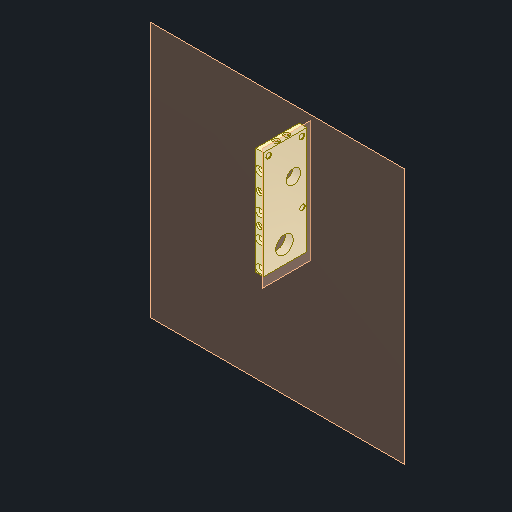
# Autodesk Inventor part: left_gear_holder
Saved by Autodesk Inventor 2023 (Build 270158000, 158)
## iProperties
Created: 2024-04-23
Part Number: left_gear_holder
Material: Nylon 6/6
Document SubType Name: Modeling
Designer: szymo
Density: 1.13 g/cm^3
Appearance: Nylon 6
Mass: 14.9327 g
Surface Area: 88.4291 cm^2
Volume: 13.2148 cm^3
Author: szymo
Autodesk Inventor part; units mm, degrees
ref_plane "YZ Plane" through (0, 0, 0) normal (1, 0, 0) x (0, 1, 0)
ref_plane "XZ Plane" through (0, 0, 0) normal (0, 1, 0) x (-1, 0, 0)
ref_plane "XY Plane" through (0, 0, 0) normal (0, 0, 1) x (1, 0, 0)
ref_plane "Work Plane1" through (0, 0, 0) normal (0, 0, 1) x (1, 0, 0)
sketch "Sketch1" plane through (0, 0, 0) normal (0, 0, 1) x (1, 0, 0)
  line L0 (23.5, 88.5) -> (-23.5, 88.5) projected
  line L1 (-23.5, 88.5) -> (-23.5, 36.5) projected
  line L2 (-26.5, 33.5) -> (-89, 33.5) projected
  line L3 (-89, 33.5) -> (-89, -72.5) projected
  line L4 (-89, -72.5) -> (-77, -72.5) projected
  line L5 (-74, -75.5) -> (-74, -93.5) projected
  line L6 (-74, -93.5) -> (74, -93.5) projected
  line L7 (74, -93.5) -> (74, -75.5) projected
  line L8 (77, -72.5) -> (89, -72.5) projected
  line L9 (89, -72.5) -> (89, 33.5) projected
  line L10 (89, 33.5) -> (26.5, 33.5) projected
  line L11 (23.5, 36.5) -> (23.5, 88.5) projected
  line L12 (-4.5, 81.5) -> (-4.5, 36.5) projected
  line L13 (-7.5, 33.5) -> (-13.5, 33.5) projected
  line L14 (-16.5, 36.5) -> (-16.5, 81.5) projected
  line L15 (-13.5, 84.5) -> (-7.5, 84.5) projected
  line L16 (16.5, 81.5) -> (16.5, 36.5) projected
  line L17 (13.5, 33.5) -> (7.5, 33.5) projected
  line L18 (4.5, 36.5) -> (4.5, 81.5) projected
  line L19 (7.5, 84.5) -> (13.5, 84.5) projected
  line L20 (16.5, 88.5) -> (22.5, 88.5)
  line L21 (22.5, 88.5) -> (22.5, 3.75)
  line L22 (22.5, 3.75) -> (16.5, 3.75)
  line L23 (16.5, 3.75) -> (16.5, 88.5)
  line L24 (59.9, 4.75) -> (32.2, 4.75)
  arc A0 (13.5, 33.5) -> (16.5, 36.5) centre (13.5, 36.5) ccw projected
  arc A1 (4.5, 36.5) -> (7.5, 33.5) centre (7.5, 36.5) ccw projected
  arc A2 (7.5, 84.5) -> (4.5, 81.5) centre (7.5, 81.5) ccw projected
  arc A3 (16.5, 81.5) -> (13.5, 84.5) centre (13.5, 81.5) ccw projected
  arc A4 (-4.5, 81.5) -> (-7.5, 84.5) centre (-7.5, 81.5) ccw projected
  arc A5 (-7.5, 33.5) -> (-4.5, 36.5) centre (-7.5, 36.5) ccw projected
  arc A6 (-16.5, 36.5) -> (-13.5, 33.5) centre (-13.5, 36.5) ccw projected
  arc A7 (-13.5, 84.5) -> (-16.5, 81.5) centre (-13.5, 81.5) ccw projected
  arc A8 (-26.5, 33.5) -> (-23.5, 36.5) centre (-26.5, 36.5) ccw projected
  arc A9 (-74, -75.5) -> (-77, -72.5) centre (-77, -75.5) ccw projected
  arc A10 (77, -72.5) -> (74, -75.5) centre (77, -75.5) ccw projected
  arc A11 (23.5, 36.5) -> (26.5, 33.5) centre (26.5, 36.5) ccw projected
  circle A12 centre (39.125, 25.9125) radius 1.0065 projected
  circle A13 centre (72.95, 12.275) radius 1.0065 projected
  circle A14 centre (-39.125, 12.3375) radius 1.0065 projected
  circle A15 centre (-72.95, 25.975) radius 1.0065 projected
  circle A16 centre (-72.95, 12.275) radius 1.0065 projected
  circle A17 centre (-39.125, 25.9125) radius 1.0065 projected
  circle A18 centre (72.95, 25.975) radius 1.0065 projected
  circle A19 centre (39.125, 12.3375) radius 1.0065 projected
  circle A20 centre (-42.4984, -44.6666) radius 1.2295 projected
  circle A21 centre (-79, -42.3889) radius 1.2295 projected
  circle A22 centre (-19.5, 28.875) radius 1.2295 projected
  circle A23 centre (19.5, 9.55) radius 1.2295 projected
  circle A24 centre (19.5, 47.3) radius 1.2295 projected
  circle A25 centre (-19.5, 47.3) radius 1.2295 projected
  circle A26 centre (0, 74.7) radius 1.2295 projected
  circle A27 centre (-19.4231, 74.8077) radius 1.2295 projected
  circle A28 centre (19.5, 74.7) radius 1.2295 projected
  circle A29 centre (0, 49.05) radius 1.2295 projected
  circle A30 centre (19.5, 28.875) radius 1.2295 projected
  circle A31 centre (0, 19.125) radius 1.2295 projected
  circle A32 centre (-19.5, 9.55) radius 1.2295 projected
  circle A33 centre (42.5, -44.6649) radius 1.2295 projected
  circle A34 centre (79, -42.3889) radius 1.2295 projected
  circle A35 centre (21.5, -85.5) radius 1.8 projected
  circle A36 centre (-64.5, -85.5) radius 1.8 projected
  circle A37 centre (-21.5, -85.5) radius 1.8 projected
  circle A38 centre (64.5, -85.5) radius 1.8 projected
  line L25 (-58.2315, -77.6013) -> (-80.7685, -61.1541) projected
  line L26 (-82, -58.7308) -> (-82, -48.3889) projected
  line L27 (-75.8885, -45.3972) -> (-47.1423, -47.5438) projected
  line L28 (-21.1, -26.5751) -> (-21.1, -22.0813) projected
  line L29 (-46.9357, -41.5592) -> (-76, -39.3889) projected
  line L30 (-82, -36.3889) -> (-82, 1.75) projected
  line L31 (32.9914, 4.75) -> (79, 4.75) projected
  line L32 (82, -48.3889) -> (82, -58.7308) projected
  line L33 (76, -39.3889) -> (46.9371, -41.5577) projected
  line L34 (21.1, -22.0813) -> (21.1, -26.5749) projected
  line L35 (47.144, -47.5423) -> (76, -45.3889) projected
  line L36 (82, 1.75) -> (82, -36.3889) projected
  line L37 (80.7685, -61.1541) -> (58.2315, -77.6013) projected
  line L38 (57, -80.0246) -> (57, -87.5) projected
  arc A39 (55, -89.5) -> (57, -87.5) centre (55, -87.5) ccw projected
  line L39 (55, -89.5) -> (31, -89.5) projected
  arc A40 (29, -87.5) -> (31, -89.5) centre (31, -87.5) ccw projected
  line L40 (29, -87.5) -> (29, -79.2522) projected
  line L41 (14, -79.5039) -> (14, -87.5) projected
  arc A41 (12, -89.5) -> (14, -87.5) centre (12, -87.5) ccw projected
  line L42 (12, -89.5) -> (-12, -89.5) projected
  arc A42 (-14, -87.5) -> (-12, -89.5) centre (-12, -87.5) ccw projected
  line L43 (-14, -87.5) -> (-14, -79.5039) projected
  line L44 (-29, -79.2522) -> (-29, -87.5) projected
  arc A43 (-31, -89.5) -> (-29, -87.5) centre (-31, -87.5) ccw projected
  line L45 (-31, -89.5) -> (-55, -89.5) projected
  arc A44 (-57, -87.5) -> (-55, -89.5) centre (-55, -87.5) ccw projected
  line L46 (-57, -87.5) -> (-57, -80.0246) projected
  line L47 (-66.95, 28.9125) -> (-45.125, 28.9125) projected
  line L48 (-42.125, 25.9125) -> (-42.125, 12.275) projected
  line L49 (-45.125, 9.275) -> (-66.95, 9.275) projected
  line L50 (-69.95, 12.275) -> (-69.95, 25.9125) projected
  line L51 (-16.5, 12.75) -> (-16.5, 25.5) projected
  line L52 (-13.5, 28.5) -> (-7.5, 28.5) projected
  line L53 (-4.5, 25.5) -> (-4.5, 12.75) projected
  line L54 (-7.5, 9.75) -> (-13.5, 9.75) projected
  line L55 (66.95, 9.3375) -> (45.125, 9.3375) projected
  line L56 (42.125, 12.3375) -> (42.125, 25.975) projected
  line L57 (45.125, 28.975) -> (66.95, 28.975) projected
  line L58 (69.95, 25.975) -> (69.95, 12.3375) projected
  line L59 (4.5, 12.75) -> (4.5, 25.5) projected
  line L60 (7.5, 28.5) -> (13.5, 28.5) projected
  line L61 (16.5, 25.5) -> (16.5, 12.75) projected
  line L62 (13.5, 9.75) -> (7.5, 9.75) projected
  line L63 (44.5181, -40.6102) -> (28.0504, -22.9209) projected
  line L64 (27.268, -20.5154) -> (30.0132, 2.1113) projected
  line L65 (-44.7206, -49.1201) -> (-29.3549, -77.8368) projected
  line L66 (-79, 4.75) -> (-32.9914, 4.75) projected
  line L67 (-30.0132, 2.1113) -> (-27.268, -20.5155) projected
  line L68 (-28.0502, -22.9208) -> (-44.5164, -40.6115) projected
  line L69 (29.3549, -77.8368) -> (44.7222, -49.1185) projected
  line L70 (-14.6042, -77.6983) -> (-37.8537, -46.8489) projected
  line L71 (-37.4786, -42.8259) -> (-22.0793, -28.7924) projected
  line L72 (-21.1218, -21.72) -> (-23.9255, 1.3887) projected
  line L73 (-20.9474, 4.75) -> (20.9474, 4.75) projected
  line L74 (23.9255, 1.3887) -> (21.1218, -21.72) projected
  line L75 (22.0795, -28.7925) -> (37.4798, -42.8243) projected
  line L76 (37.8551, -46.8475) -> (14.6042, -77.6983) projected
  circle A45 centre (-78, -67.1725) radius 1.2295 projected
  arc A46 (79, -39.3889) -> (82, -36.3889) centre (79, -36.3889) ccw projected
  arc A47 (44.5181, -40.6102) -> (46.9371, -41.5577) centre (46.7138, -38.566) ccw projected
  arc A48 (27.268, -20.5154) -> (28.0504, -22.9209) centre (30.2461, -20.8767) ccw projected
  arc A49 (32.9914, 4.75) -> (30.0132, 2.1113) centre (32.9914, 1.75) ccw projected
  arc A50 (82, 1.75) -> (79, 4.75) centre (79, 1.75) ccw projected
  arc A51 (-42.125, 25.9125) -> (-45.125, 28.9125) centre (-45.125, 25.9125) ccw projected
  arc A52 (-45.125, 9.275) -> (-42.125, 12.275) centre (-45.125, 12.275) ccw projected
  arc A53 (-69.95, 12.275) -> (-66.95, 9.275) centre (-66.95, 12.275) ccw projected
  arc A54 (-66.95, 28.9125) -> (-69.95, 25.9125) centre (-66.95, 25.9125) ccw projected
  arc A55 (-13.5, 28.5) -> (-16.5, 25.5) centre (-13.5, 25.5) ccw projected
  arc A56 (-4.5, 25.5) -> (-7.5, 28.5) centre (-7.5, 25.5) ccw projected
  arc A57 (-7.5, 9.75) -> (-4.5, 12.75) centre (-7.5, 12.75) ccw projected
  arc A58 (-16.5, 12.75) -> (-13.5, 9.75) centre (-13.5, 12.75) ccw projected
  arc A59 (58.2315, -77.6013) -> (57, -80.0246) centre (60, -80.0246) ccw projected
  arc A60 (29.3549, -77.8368) -> (29, -79.2522) centre (32, -79.2522) ccw projected
  arc A61 (47.144, -47.5423) -> (44.7222, -49.1185) centre (47.3673, -50.5339) ccw projected
  arc A62 (82, -48.3889) -> (79, -45.3889) centre (79, -48.3889) ccw projected
  arc A63 (80.7685, -61.1541) -> (82, -58.7308) centre (79, -58.7308) ccw projected
  arc A64 (-21.1, -22.0813) -> (-21.1218, -21.72) centre (-24.1, -22.0813) ccw projected
  arc A65 (-20.9474, 4.75) -> (-23.9255, 1.3887) centre (-20.9474, 1.75) ccw projected
  arc A66 (23.9255, 1.3887) -> (20.9474, 4.75) centre (20.9474, 1.75) ccw projected
  arc A67 (21.1218, -21.72) -> (21.1, -22.0813) centre (24.1, -22.0813) ccw projected
  arc A68 (21.1, -26.5749) -> (22.0795, -28.7925) centre (24.1, -26.5749) ccw projected
  arc A69 (37.8551, -46.8475) -> (37.4798, -42.8243) centre (35.4593, -45.0419) ccw projected
  arc A70 (14.6042, -77.6983) -> (14, -79.5039) centre (17, -79.5039) ccw projected
  arc A71 (-14, -79.5039) -> (-14.6042, -77.6983) centre (-17, -79.5039) ccw projected
  arc A72 (-37.4786, -42.8259) -> (-37.8537, -46.8489) centre (-35.4579, -45.0433) ccw projected
  arc A73 (-22.0793, -28.7924) -> (-21.1, -26.5751) centre (-24.1, -26.5751) ccw projected
  arc A74 (-82, -36.3889) -> (-79, -39.3889) centre (-79, -36.3889) ccw projected
  arc A75 (-79, 4.75) -> (-82, 1.75) centre (-79, 1.75) ccw projected
  arc A76 (-30.0132, 2.1113) -> (-32.9914, 4.75) centre (-32.9914, 1.75) ccw projected
  arc A77 (-28.0502, -22.9208) -> (-27.268, -20.5155) centre (-30.2461, -20.8769) ccw projected
  arc A78 (-46.9357, -41.5592) -> (-44.5164, -40.6115) centre (-46.7123, -38.5676) ccw projected
  arc A79 (7.5, 28.5) -> (4.5, 25.5) centre (7.5, 25.5) ccw projected
  arc A80 (16.5, 25.5) -> (13.5, 28.5) centre (13.5, 25.5) ccw projected
  arc A81 (13.5, 9.75) -> (16.5, 12.75) centre (13.5, 12.75) ccw projected
  arc A82 (4.5, 12.75) -> (7.5, 9.75) centre (7.5, 12.75) ccw projected
  arc A83 (-57, -80.0246) -> (-58.2315, -77.6013) centre (-60, -80.0246) ccw projected
  arc A84 (-82, -58.7308) -> (-80.7685, -61.1541) centre (-79, -58.7308) ccw projected
  arc A85 (-75.8885, -45.3972) -> (-76.1119, -45.3889) centre (-76.1119, -48.3889) ccw projected
  arc A86 (-44.7206, -49.1201) -> (-47.1423, -47.5438) centre (-47.3657, -50.5355) ccw projected
  arc A87 (-29, -79.2522) -> (-29.3549, -77.8368) centre (-32, -79.2522) ccw projected
  arc A88 (42.125, 12.3375) -> (45.125, 9.3375) centre (45.125, 12.3375) ccw projected
  arc A89 (45.125, 28.975) -> (42.125, 25.975) centre (45.125, 25.975) ccw projected
  arc A90 (69.95, 25.975) -> (66.95, 28.975) centre (66.95, 25.975) ccw projected
  arc A91 (66.95, 9.3375) -> (69.95, 12.3375) centre (66.95, 12.3375) ccw projected
  circle A92 centre (78, -67.1725) radius 1.2295 projected
  line L77 (-22.5, 25.9125) -> (-22.5, 12.55) projected
  arc A93 (-25.5, 9.55) -> (-22.5, 12.55) centre (-25.5, 12.55) ccw projected
  line L78 (-25.5, 9.55) -> (-33.125, 9.55) projected
  arc A94 (-36.125, 12.55) -> (-33.125, 9.55) centre (-33.125, 12.55) ccw projected
  line L79 (-36.125, 12.55) -> (-36.125, 25.9125) projected
  arc A95 (-33.125, 28.9125) -> (-36.125, 25.9125) centre (-33.125, 25.9125) ccw projected
  line L80 (-33.125, 28.9125) -> (-25.5, 28.9125) projected
  arc A96 (-22.5, 25.9125) -> (-25.5, 28.9125) centre (-25.5, 25.9125) ccw projected
  line L81 (76, -45.3889) -> (79, -45.3889) projected
  line L82 (79, -39.3889) -> (76, -39.3889) projected
  line L83 (33.125, 9.275) -> (25.5, 9.275) projected
  arc A97 (22.5, 12.275) -> (25.5, 9.275) centre (25.5, 12.275) ccw projected
  line L84 (22.5, 12.275) -> (22.5, 25.9125) projected
  arc A98 (25.5, 28.9125) -> (22.5, 25.9125) centre (25.5, 25.9125) ccw projected
  line L85 (25.5, 28.9125) -> (33.125, 28.9125) projected
  arc A99 (36.125, 25.9125) -> (33.125, 28.9125) centre (33.125, 25.9125) ccw projected
  line L86 (36.125, 25.9125) -> (36.125, 12.275) projected
  arc A100 (33.125, 9.275) -> (36.125, 12.275) centre (33.125, 12.275) ccw projected
  line L87 (-83, 28.975) -> (-78.95, 28.975) projected
  arc A101 (-75.95, 25.975) -> (-78.95, 28.975) centre (-78.95, 25.975) ccw projected
  line L88 (-75.95, 25.975) -> (-75.95, 12.275) projected
  arc A102 (-78.95, 9.275) -> (-75.95, 12.275) centre (-78.95, 12.275) ccw projected
  line L89 (-78.95, 9.275) -> (-83, 9.275) projected
  arc A103 (-86, 12.275) -> (-83, 9.275) centre (-83, 12.275) ccw projected
  line L90 (-86, 12.275) -> (-86, 25.975) projected
  arc A104 (-83, 28.975) -> (-86, 25.975) centre (-83, 25.975) ccw projected
  arc A105 (-79, -45.3889) -> (-82, -48.3889) centre (-79, -48.3889) ccw projected
  line L91 (-79, -45.3889) -> (-76.1119, -45.3889) projected
  line L92 (-76, -39.3889) -> (-79, -39.3889) projected
  line L93 (78.95, 28.975) -> (83, 28.975) projected
  arc A106 (86, 25.975) -> (83, 28.975) centre (83, 25.975) ccw projected
  line L94 (86, 25.975) -> (86, 12.275) projected
  arc A107 (83, 9.275) -> (86, 12.275) centre (83, 12.275) ccw projected
  line L95 (83, 9.275) -> (78.95, 9.275) projected
  arc A108 (75.95, 12.275) -> (78.95, 9.275) centre (78.95, 12.275) ccw projected
  line L96 (75.95, 12.275) -> (75.95, 25.975) projected
  arc A109 (78.95, 28.975) -> (75.95, 25.975) centre (78.95, 25.975) ccw projected
  circle A110 centre (-24.1, -73.1) radius 1.2295 projected
  circle A111 centre (24.1, -24.9) radius 1.2295 projected
  circle A112 centre (-24.1, -24.9) radius 1.2295 projected
  circle A113 centre (24.1, -73.1) radius 1.2295 projected
  point P0 (0, 0)
  point P1 (7.5, 81.5)
  point P2 (13.5, 81.5)
  point P3 (-7.5, 81.5)
  point P4 (-13.5, 81.5)
  point P5 (-77, -75.5)
  point P6 (39, -44.2094)
  point P7 (16.5, 28.5)
  point P8 (16.5, 9.75)
  point P9 (-79, -67.8878)
  point P10 (-79, -66.4572)
  dimension "d0" = 1
  dimension "d1" = 1
  constraints: 10 end point, 2 horizontal, 2 parallel, 1 collinear, 1 perpendicular, 1 point on line, 2 other
  measures "d0" distance between parallel lines of L21 L11
  measures "d1" distance between parallel lines of L24 L22
ref_plane "Work Plane2" through (-89, -40.3889, 33.5) normal (0, 0, 1) x (1, 0, 0)
extrude "Extrusion1" add sketch "Sketch1" along normal up to surface (33.5 mm away) contours L21 A66 L73 L23 L16 L0 | L21 L22 L23 L73 A66 | A23 | A24 | A28 | A30
sketch "Sketch2" plane through (22.5, 3.75, 0) normal (1, 0, 0) x (0, 0, -1)
  circle A0 centre (-17.375, 15.375) radius 6.75 projected
  circle A1 centre (-10.5, 57.25) radius 5.5 projected
  point P0 (0, -3.75)
  dimension "d8" = 11
  measures "d8" diameter of A1
extrude "Extrusion2" cut sketch "Sketch2" against normal up to next
sketch "Sketch3" plane through (16.5, 3.75, 0) normal (-1, 0, 0) x (0, 0, 1)
  circle A0 centre (23.4363, 30.1825) radius 2 projected
  point P0 (0, -3.75)
extrude "Extrusion3" cut sketch "Sketch3" against normal blind 5
ref_plane "Work Plane3" through (23.5, 3.75, 0) normal (1, 0, 0) x (0, 0, -1)
sketch "Sketch4" plane through (23.5, 3.75, 0) normal (1, 0, 0) x (0, 0, -1)
  circle A0 centre (-29.5, 80.75) radius 1.8 projected
  circle A1 centre (-3.5, 33.25) radius 1.8 projected
  circle A2 centre (-4, 80.75) radius 1.8 projected
  point P0 (0, -3.75)
hole "Hole1" at (23.5, 37, 3.5) at (23.5, 84.5, 4) at (23.5, 84.5, 29.5) direction (-1, 0, 0) diameter 3.6 end through all countersink diameter 6.2 countersink angle 90 clearance for "Countersunk Flat Head Screw ISO 2009/7046" size "M3" standard "ISO"
sketch "Sketch5" plane through (16.5, 3.75, 33.5) normal (0, 0, 1) x (1, 0, 0)
  circle A0 centre (-36, 5.8) radius 1.8 projected
  circle A1 centre (-36, 25.125) radius 1.8 projected
  circle A2 centre (-36, 43.55) radius 1.8 projected
  circle A3 centre (-35.9231, 71.0577) radius 1.8 projected
  circle A4 centre (-16.5, 45.3) radius 3.3 projected
  circle A5 centre (-16.5, 15.375) radius 3.3 projected
  circle A6 centre (-16.5, 70.95) radius 3.3 projected
  line L0 (-12, 2) -> (-21, 2) projected
  line L1 (-12, 84.75) -> (-12, 2) projected
  line L2 (-21, 84.75) -> (-12, 84.75) projected
  line L3 (-21, 2) -> (-21, 84.75) projected
  line L4 (-16.5, 2) -> (-16.5, 84.75)
  circle A7 centre (3, 5.8) radius 1.8
  circle A8 centre (3, 25.125) radius 1.8
  circle A9 centre (3, 43.55) radius 1.8
  circle A10 centre (2.9231, 71.0577) radius 1.8
  circle A11 centre (-16.5, 30.7161) radius 2.3 projected
  circle A12 centre (-16.5, 59.25) radius 2.3 projected
  point P0 (-16.5, -3.75)
  constraints: 4 centre point, 4 coincident, 4 symmetric about line, 2 end point, 2 midpoint, 4 other
hole "Hole2" at (19.5, 9.55, 33.5) at (19.5, 28.875, 33.5) at (19.5, 47.3, 33.5) at (19.4231, 74.8077, 33.5) direction (0, 0, -1) diameter 3.6 end through all countersink diameter 6.3 countersink angle 90 clearance for "Countersunk Flat Head Screw ISO 2009/7046" size "M3" standard "ISO"
sketch "Sketch7" plane through (16.5, 88.5, 0) normal (0, 1, 0) x (1, 0, 0)
  line L0 (0, -33.5) -> (6, -33.5) projected
  line L1 (6, 0) -> (6, -33.5) projected
  line L2 (6, 0) -> (0, 0) projected
  line L3 (0, 0) -> (0, -33.5) projected
  circle A0 centre (-16.5, -12.675) radius 2 projected
  circle A1 centre (-16.5, -20.825) radius 2 projected
  line L4 (-16.5, -20.825) -> (6, -20.825)
  line L5 (-16.5, -12.675) -> (6, -12.675)
  line L6 (6, -5) -> (6, -16) projected
  point P0 (-16.5, 0)
  point P1 (3, -20.825)
  point P2 (3, -12.675)
  constraints: 4 end point, 4 point on line, 2 perpendicular
hole "Hole4" at (19.5, 88.5, 20.825) at (19.5, 88.5, 12.675) direction (0, -1, 0) diameter 4 depth 6 counterbore diameter 4.6 counterbore depth 1.5
sketch "Sketch8" plane through (19.5, 47.3, 33.5) normal (0, 0, 1) x (1, 0, 0)
  circle A0 centre (-39, -9.2125) radius 2.3 projected
  circle A1 centre (-39, 13.7) radius 2.3 projected
  arc A2 (3, 0.9605) -> (-3, 0.9605) centre (0, 0) ccw projected
  line L0 (3, 26.8331) -> (3, 0.9605) projected
  arc A3 (-3, 26.3338) -> (3, 26.8331) centre (-0.0769, 27.5077) ccw projected
  line L1 (-3, 0.9605) -> (-3, 26.3338) projected
  arc A4 (-3, -0.9605) -> (3, -0.9605) centre (0, 0) ccw projected
  line L2 (-3, -17.4645) -> (-3, -0.9605) projected
  arc A5 (3, -17.4645) -> (-3, -17.4645) centre (0, -18.425) ccw projected
  line L3 (3, -0.9605) -> (3, -17.4645) projected
  line L4 (-39, 13.7) -> (3, 13.7)
  line L5 (3, 19.2) -> (3, 8.2) projected
  line L6 (-39, -9.2125) -> (3, -9.2125)
  circle A6 centre (0, -18.425) radius 1.8 projected
  line L7 (0, -18.425) -> (-0.0769, 27.5077)
  point P0 (-19.5, -47.3)
  point P1 (-0.0538, 13.7)
  point P2 (-0.0154, -9.2125)
  constraints: 6 end point, 4 point on line, 2 midpoint
hole "Hole5" at (19.4462, 61, 33.5) at (19.4846, 38.0875, 33.5) direction (0, 0, -1) diameter 4 depth 6 counterbore diameter 4.6 counterbore depth 1.5
sketch "Sketch9" plane through (16.5, 3.75, 0) normal (0, -1, 0) x (1, 0, 0)
  line L0 (0, 0) -> (0, 33.5) projected
  line L1 (0, 0) -> (6, 0) projected
  line L2 (6, 0) -> (6, 33.5) projected
  line L3 (6, 33.5) -> (0, 33.5) projected
  point P0 (-16.5, 0)
extrude "Extrusion4" cut sketch "Sketch9" against normal blind 2
body "Solid1"
